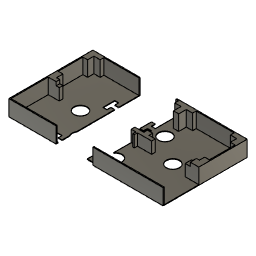
loose_split (Autodesk Fusion 360 design; units mm, degrees)
Autodesk Fusion 360 part; units mm, degrees
note: some values were not read from the file. Chosen so that the rebuilt part matches the saved one: which face or edge a step refers to. Set by a fixed rule: which sketch regions a step uses.
(part 1 of 2)
sketch "スケッチ1" plane through (0, 0, 0) normal (0, 0, 1) x (1, 0, 0)
  line L0 (0, 0) -> (224, 0)
  line L1 (224, 0) -> (224, 158)
  line L2 (224, 158) -> (0, 158)
  line L3 (0, 158) -> (0, 0)
  dimension "d1" = 224
  dimension "d2" = 158
  constraint horizontal L0
  constraint vertical L1
  constraint horizontal L2
  constraint vertical L3
  constraint coincident L0.start L3.end
  measures "d1" distance of L0.start L0.end
  measures "d2" distance of L0.start L2.end
extrude "押し出し1" add sketch "スケッチ1" along normal blind 30 makes body 1
sketch "スケッチ2" plane through (0, 0, 30) normal (0, 0, 1) x (-1, 0, 0)
  line L0 (0, -158) -> (0, 0)
  line L1 (0, 0) -> (-224, 0)
  line L2 (-224, 0) -> (-224, -158)
  line L3 (-224, -158) -> (0, -158)
  line L4 (0, 0) -> (-2, 0)
  line L5 (-2, 0) -> (-2, -2)
  line L6 (-2, -2) -> (0, -2)
  line L7 (0, -2) -> (0, 0)
  line L8 (-224, -158) -> (-222, -158)
  line L9 (-222, -158) -> (-222, -156)
  line L10 (-222, -156) -> (-224, -156)
  line L11 (-224, -156) -> (-224, -158)
  dimension "d5" = 2
  dimension "d6" = 2
  dimension "d7" = 2
  dimension "d8" = 2
  constraint horizontal L4
  constraint vertical L5
  constraint horizontal L6
  constraint vertical L7
  constraint coincident L0.end L1.start
  constraint horizontal L8
  constraint vertical L9
  constraint horizontal L10
  constraint vertical L11
  constraint coincident L2.end L3.start
  measures "d5" distance of L0.end L4.end
  measures "d6" distance of L0.end L6.end
  measures "d7" distance of L2.end L8.end
  measures "d8" distance of L2.end L10.end
sketch "スケッチ3" plane through (0, 0, 30) normal (0, 0, 1) x (-1, 0, 0)
  line L0 (-2, -2) -> (-222, -2)
  line L1 (-222, -2) -> (-222, -156)
  line L2 (-222, -156) -> (-2, -156)
  line L3 (-2, -156) -> (-2, -2)
  point P0 (-2, -2)
  point P1 (-222, -156)
  constraint horizontal L0
  constraint vertical L1
  constraint horizontal L2
  constraint vertical L3
  constraint coincident P1 L1.end
  constraint coincident P0 L0.start
extrude "押し出し2" cut sketch "スケッチ3" against normal blind 28 bodies 1
sketch "スケッチ4" plane through (0, 0, 2) normal (0, 0, 1) x (-1, 0, 0)
  line L0 (-2, -156) -> (-2, -2)
  line L1 (-2, -2) -> (-222, -2)
  line L2 (-222, -2) -> (-222, -156)
  line L3 (-222, -156) -> (-2, -156)
sketch "スケッチ14" plane through (0, 0, 30) normal (0, 0, 1) x (-1, 0, 0)
  line L0 (-222, -2) -> (-2, -2)
  line L1 (-2, -2) -> (-2, -156)
  line L2 (-2, -156) -> (-222, -156)
  line L3 (-222, -156) -> (-222, -2)
  line L4 (0, -158) -> (0, 0)
  line L5 (0, 0) -> (-224, 0)
  line L6 (-224, 0) -> (-224, -158)
  line L7 (-224, -158) -> (0, -158)
sketch "スケッチ15" plane through (0, 0, 30) normal (0, 0, 1) x (-1, 0, 0)
  line L0 (-224, -2) -> (-99, -2)
  line L1 (-99, -2) -> (-99, -66)
  line L2 (-99, -66) -> (-224, -66)
  line L3 (-224, -66) -> (-224, -2)
  line L4 (-224, 0) -> (-224, -158)
  dimension "d41" = 125
  dimension "d42" = 64
  constraint horizontal L0
  constraint vertical L1
  constraint horizontal L2
  constraint vertical L3
  constraint coincident L0.start L4
  measures "d41" distance of L0.start L0.end
  measures "d42" distance of L0.start L2.end
extrude "押し出し10" cut sketch "スケッチ15" against normal blind 29 bodies 1
sketch "スケッチ16" plane through (0, 0, 30) normal (0, 0, 1) x (-1, 0, 0)
  line L0 (-2, -2) -> (-99, -2)
  line L1 (-99, -2) -> (-99, -73)
  line L2 (-99, -73) -> (-2, -73)
  line L3 (-2, -73) -> (-2, -2)
  point P0 (-2, -2)
  dimension "d45" = 71
  constraint horizontal L0
  constraint vertical L1
  constraint horizontal L2
  constraint vertical L3
  constraint coincident P0 L0.start
  measures "d45" distance of P0 L2.end
extrude "押し出し11" add 1 faces at (182.3333, 23.3333, 1) along direction (0, 0, 1) blind 1 on bodies 1 bodies 1
sketch "スケッチ17" plane through (0, 0, 30) normal (0, 0, 1) x (1, 0, 0)
  line L0 (2, 156) -> (11, 156)
  line L1 (11, 156) -> (11, 147)
  line L2 (11, 147) -> (2, 147)
  line L3 (2, 147) -> (2, 156)
  line L4 (11, 147) -> (107, 147)
  line L5 (107, 147) -> (107, 76)
  line L6 (107, 76) -> (11, 76)
  line L7 (11, 76) -> (11, 147)
  line L8 (222, 156) -> (213, 156)
  line L9 (213, 156) -> (213, 147)
  line L10 (213, 147) -> (222, 147)
  line L11 (222, 147) -> (222, 156)
  line L12 (213, 147) -> (117, 147)
  line L13 (117, 147) -> (117, 76)
  line L14 (117, 76) -> (213, 76)
  line L15 (213, 76) -> (213, 147)
  point P0 (2, 156)
  point P1 (222, 156)
  dimension "d48" = 9
  dimension "d49" = 9
  dimension "d50" = 96
  dimension "d51" = 71
  dimension "d52" = 9
  dimension "d53" = 9
  dimension "d54" = 96
  dimension "d55" = 71
  constraint horizontal L0
  constraint vertical L1
  constraint horizontal L2
  constraint vertical L3
  constraint coincident P0 L0.start
  constraint horizontal L4
  constraint vertical L5
  constraint horizontal L6
  constraint vertical L7
  constraint horizontal L8
  constraint vertical L9
  constraint horizontal L10
  constraint vertical L11
  constraint coincident P1 L8.start
  constraint horizontal L12
  constraint vertical L13
  constraint horizontal L14
  constraint vertical L15
  measures "d48" distance of P0 L0.end
  measures "d49" distance of P0 L2.end
  measures "d50" distance of L1.end L4.end
  measures "d51" distance of L1.end L6.end
  measures "d52" distance of P1 L8.end
  measures "d53" distance of P1 L10.end
  measures "d54" distance of L9.end L12.end
  measures "d55" distance of L9.end L14.end
sketch "スケッチ18" plane through (0, 0, 30) normal (0, 0, 1) x (-1, 0, 0)
  line L0 (-11, -147) -> (-2, -147)
  line L1 (-2, -147) -> (-2, -138)
  line L2 (-2, -138) -> (-11, -138)
  line L3 (-11, -138) -> (-11, -147)
  line L4 (-11, -147) -> (-20, -147)
  line L5 (-20, -147) -> (-20, -156)
  line L6 (-20, -156) -> (-11, -156)
  line L7 (-11, -156) -> (-11, -147)
  point P0 (-11, -147)
  dimension "d56" = 9
  dimension "d57" = 9
  dimension "d58" = 9
  constraint horizontal L0
  constraint vertical L1
  constraint horizontal L2
  constraint vertical L3
  constraint coincident P0 L0.start
  constraint horizontal L4
  constraint vertical L5
  constraint horizontal L6
  constraint vertical L7
  measures "d56" distance of P0 L0.end
  measures "d57" distance of P0 L2.end
  measures "d58" distance of P0 L6.end
extrude "押し出し12" add sketch "スケッチ17" sketch "スケッチ18" against normal blind 28 contours L0 L1 L2 L3 of sketch 2 bodies 1
sketch "スケッチ19" plane through (0, 0, 2) normal (0, 0, 1) x (-1, 0, 0)
  line L0 (-213, -147) -> (-222, -147)
  line L1 (-222, -147) -> (-222, -138)
  line L2 (-222, -138) -> (-213, -138)
  line L3 (-213, -138) -> (-213, -147)
  line L4 (-213, -147) -> (-204, -147)
  line L5 (-204, -147) -> (-204, -156)
  line L6 (-204, -156) -> (-213, -156)
  line L7 (-213, -156) -> (-213, -147)
  point P0 (-213, -147)
  dimension "d61" = 9
  dimension "d62" = 9
  dimension "d63" = 9
  dimension "d64" = 9
  constraint horizontal L0
  constraint vertical L1
  constraint horizontal L2
  constraint vertical L3
  constraint coincident P0 L0.start
  constraint horizontal L4
  constraint vertical L5
  constraint horizontal L6
  constraint vertical L7
  measures "d61" distance of P0 L0.end
  measures "d62" distance of P0 L2.end
  measures "d63" distance of P0 L4.end
  measures "d64" distance of P0 L6.end
extrude "押し出し13" add sketch "スケッチ19" along normal blind 28 separate body makes body 2 at (210, 147, 11.3333)
extrude "押し出し14" add sketch "スケッチ17" against normal blind 28 contours L8 L9 L10 L11 bodies 1 2
sketch "スケッチ20" plane through (0, 0, 2) normal (0, 0, 1) x (-1, 0, 0)
  line L0 (-107, -147) -> (-117, -147)
  line L1 (-117, -147) -> (-117, -138)
  line L2 (-117, -138) -> (-107, -138)
  line L3 (-107, -138) -> (-107, -147)
  line L4 (-107, -147) -> (-98, -147)
  line L5 (-98, -147) -> (-98, -156)
  line L6 (-98, -156) -> (-107, -156)
  line L7 (-107, -156) -> (-107, -147)
  line L8 (-117, -147) -> (-126, -147)
  line L9 (-126, -147) -> (-126, -156)
  line L10 (-126, -156) -> (-117, -156)
  line L11 (-117, -156) -> (-117, -147)
  line L12 (-99, -66) -> (-126, -66)
  line L13 (-126, -66) -> (-126, -76)
  line L14 (-126, -76) -> (-99, -76)
  line L15 (-99, -76) -> (-99, -66)
  line L16 (-107, -76) -> (-117, -76)
  line L17 (-117, -76) -> (-117, -85)
  line L18 (-117, -85) -> (-107, -85)
  line L19 (-107, -85) -> (-107, -76)
  point P0 (-107, -147)
  point P1 (-99, -66)
  point P2 (-107, -76)
  dimension "d69" = 10
  dimension "d70" = 9
  dimension "d71" = 9
  dimension "d72" = 9
  dimension "d73" = 9
  dimension "d74" = 9
  dimension "d75" = 27
  dimension "d76" = 9
  constraint horizontal L0
  constraint vertical L1
  constraint horizontal L2
  constraint vertical L3
  constraint coincident P0 L0.start
  constraint horizontal L4
  constraint vertical L5
  constraint horizontal L6
  constraint vertical L7
  constraint horizontal L8
  constraint vertical L9
  constraint horizontal L10
  constraint vertical L11
  constraint horizontal L12
  constraint vertical L13
  constraint horizontal L14
  constraint vertical L15
  constraint coincident P1 L12.start
  constraint horizontal L16
  constraint vertical L17
  constraint horizontal L18
  constraint vertical L19
  constraint coincident P2 L16.start
  measures "d69" distance of P0 L0.end
  measures "d70" distance of P0 L2.end
  measures "d71" distance of P0 L4.end
  measures "d72" distance of P0 L6.end
  measures "d73" distance of L0.end L8.end
  measures "d74" distance of L0.end L10.end
  measures "d75" distance of P1 L12.end
  measures "d76" distance of P2 L18.end
extrude "押し出し15" add sketch "スケッチ20" along normal blind 28 separate body contours L8 L9 L10 L11 | L0 L1 L2 L3 | L4 L5 L6 L7 makes body 3 at (104, 147, 11.3333)
extrude "押し出し16" add 1 faces at (110.3333, 147, 11.3333) along direction (0, 1, 0) blind 9 on bodies 3 bodies 1 3
extrude "押し出し17" add sketch "スケッチ20" along normal blind 28 contours L12 L13 L14 L15 L16 | L14 L16 L17 L18 L19 bodies 1
sketch "スケッチ21" plane through (0, 0, 2) normal (0, 0, 1) x (-1, 0, 0)
  line L0 (-99, -76) -> (-90, -76)
  line L1 (-90, -76) -> (-90, -73)
  line L2 (-90, -73) -> (-99, -73)
  line L3 (-99, -73) -> (-99, -76)
  point P0 (-99, -76)
  dimension "d83" = 9
  constraint horizontal L0
  constraint vertical L1
  constraint horizontal L2
  constraint vertical L3
  constraint coincident P0 L0.start
  measures "d83" distance of P0 L0.end
extrude "押し出し18" add sketch "スケッチ21" along normal blind 28 bodies 1
sketch "スケッチ22" plane through (0, 0, 2) normal (0, 0, 1) x (-1, 0, 0)
  line L0 (-11, -76) -> (-20, -76)
  line L1 (-20, -76) -> (-20, -73)
  line L2 (-20, -73) -> (-11, -73)
  line L3 (-11, -73) -> (-11, -76)
  line L4 (-11, -73) -> (-2, -73)
  line L5 (-2, -73) -> (-2, -85)
  line L6 (-2, -85) -> (-11, -85)
  line L7 (-11, -85) -> (-11, -73)
  point P0 (-11, -76)
  dimension "d86" = 9
  dimension "d87" = 3
  dimension "d88" = 12
  constraint horizontal L0
  constraint vertical L1
  constraint horizontal L2
  constraint vertical L3
  constraint coincident P0 L0.start
  constraint horizontal L4
  constraint vertical L5
  constraint horizontal L6
  constraint vertical L7
  measures "d86" distance of P0 L0.end
  measures "d87" distance of P0 L2.end
  measures "d88" distance of L2.end L6.end
extrude "押し出し19" add sketch "スケッチ22" along normal blind 28 bodies 1
sketch "スケッチ23" plane through (0, 0, 2) normal (0, 0, 1) x (-1, 0, 0)
  line L0 (-213, -76) -> (-204, -76)
  line L1 (-204, -76) -> (-204, -66)
  line L2 (-204, -66) -> (-213, -66)
  line L3 (-213, -66) -> (-213, -76)
  line L4 (-213, -76) -> (-222, -76)
  line L5 (-222, -76) -> (-222, -85)
  line L6 (-222, -85) -> (-213, -85)
  line L7 (-213, -85) -> (-213, -76)
  line L8 (-213, -76) -> (-222, -76)
  line L9 (-222, -76) -> (-222, -66)
  line L10 (-222, -66) -> (-213, -66)
  line L11 (-213, -66) -> (-213, -76)
  point P0 (-213, -76)
  point P1 (-222, -66)
  dimension "d91" = 9
  dimension "d92" = 9
  dimension "d93" = 9
  constraint horizontal L0
  constraint vertical L1
  constraint horizontal L2
  constraint vertical L3
  constraint coincident P0 L0.start
  constraint horizontal L4
  constraint vertical L5
  constraint horizontal L6
  constraint vertical L7
  constraint horizontal L8
  constraint vertical L9
  constraint horizontal L10
  constraint vertical L11
  constraint coincident P1 L9.end
  measures "d91" distance of P0 L0.end
  measures "d92" distance of P0 L4.end
  measures "d93" distance of P0 L6.end
extrude "押し出し20" add sketch "スケッチ23" along normal blind 28 bodies 1
sketch "スケッチ24" plane through (0, 0, 30) normal (0, 0, 1) x (-1, 0, 0)
  line L0 (-107, -138) -> (-117, -138)
  line L1 (-117, -138) -> (-117, -147)
  line L2 (-117, -147) -> (-126, -147)
  line L3 (-126, -147) -> (-126, -156)
  line L4 (-126, -156) -> (-204, -156)
  line L5 (-204, -156) -> (-204, -147)
  line L6 (-204, -147) -> (-213, -147)
  line L7 (-213, -147) -> (-213, -138)
  line L8 (-213, -138) -> (-222, -138)
  line L9 (-222, -138) -> (-222, -85)
  line L10 (-222, -85) -> (-213, -85)
  line L11 (-213, -85) -> (-213, -76)
  line L12 (-213, -76) -> (-204, -76)
  line L13 (-204, -76) -> (-204, -66)
  line L14 (-204, -66) -> (-224, -66)
  line L15 (-224, -66) -> (-224, -158)
  line L16 (-224, -158) -> (0, -158)
  line L17 (0, -158) -> (0, 0)
  line L18 (0, 0) -> (-224, 0)
  line L19 (-224, 0) -> (-224, -2)
  line L20 (-224, -2) -> (-2, -2)
  line L21 (-2, -2) -> (-2, -73)
  line L22 (-2, -73) -> (-20, -73)
  line L23 (-20, -73) -> (-20, -76)
  line L24 (-20, -76) -> (-11, -76)
  line L25 (-11, -76) -> (-11, -85)
  line L26 (-11, -85) -> (-2, -85)
  line L27 (-2, -85) -> (-2, -138)
  line L28 (-2, -138) -> (-11, -138)
  line L29 (-11, -138) -> (-11, -147)
  line L30 (-11, -147) -> (-20, -147)
  line L31 (-20, -147) -> (-20, -156)
  line L32 (-20, -156) -> (-98, -156)
  line L33 (-98, -156) -> (-98, -147)
  line L34 (-98, -147) -> (-107, -147)
  line L35 (-107, -147) -> (-107, -138)
  line L36 (-2, -156) -> (-222, -156)
  line L37 (-222, -156) -> (-222, -2)
  line L38 (-222, -2) -> (-2, -2)
  line L39 (-2, -2) -> (-2, -156)
  point P0 (-2, -156)
  point P1 (-222, -2)
  constraint horizontal L36
  constraint vertical L37
  constraint horizontal L38
  constraint vertical L39
  constraint coincident P1 L37.end
  constraint coincident P0 L36.start
extrude "押し出し21" cut sketch "スケッチ24" against normal blind 7 contours L0 L1 L2 L3 L33 L34 L35 L36 | L0 L1 L2 L3 L4 L5 L6 L7 L8 L9 L10 L11 L12 L13 L14 L20 L21 L22 L23 L24 L25 L26 L27 L28 L29 L30 L31 L32 L33 L34 L35 L36 L37 L38 L39 | L28 L29 L30 L31 L36 L39 | L5 L6 L7 L8 L36 L37 | L22 L23 L24 L25 L26 L39 | L10 L11 L12 L13 L14 L37 bodies 1
sketch "スケッチ25" plane through (0, 0, 30) normal (0, 0, 1) x (1, 0, 0)
  line L0 (90, 73) -> (85, 73)
  line L1 (85, 73) -> (85, -7.0693)
  line L2 (85, -7.0693) -> (90, -7.0693)
  line L3 (90, -7.0693) -> (90, 73)
  line L4 (90, 73) -> (85, 73)
  line L5 (85, 73) -> (85, 169.9061)
  line L6 (85, 169.9061) -> (90, 169.9061)
  line L7 (90, 169.9061) -> (90, 73)
  point P0 (90, 73)
  dimension "d98" = 5
  dimension "d99" = 5
  constraint horizontal L0
  constraint vertical L1
  constraint horizontal L2
  constraint vertical L3
  constraint coincident P0 L0.start
  constraint horizontal L4
  constraint vertical L5
  constraint horizontal L6
  constraint vertical L7
  measures "d98" distance of P0 L0.end
  measures "d99" distance of P0 L0.end
extrude "押し出し22" cut sketch "スケッチ25" against normal blind 70 bodies 1 makes body 4 at (28.3333, 105.3333, 0)
move_body "移動1" bodies 1 to x (1, 0, 0) y (0, 1, 0) z (0, 0, 1) at (70, 0, 0)
extrude "押し出し23" add 1 faces at (85, 53.3333, 0.6667) along direction (1, 0, 0) blind 5 on bodies 4 bodies 4
sketch "スケッチ26" plane through (0, 0, 2) normal (0, 0, 1) x (-1, 0, 0)
  line L0 (-90, -156) -> (-20, -156)
  line L1 (-20, -156) -> (-20, -147)
  line L2 (-20, -147) -> (-11, -147)
  line L3 (-11, -147) -> (-11, -138)
  line L4 (-11, -138) -> (-2, -138)
  line L5 (-2, -138) -> (-2, -85)
  line L6 (-2, -85) -> (-11, -85)
  line L7 (-11, -85) -> (-11, -76)
  line L8 (-11, -76) -> (-20, -76)
  line L9 (-20, -76) -> (-20, -73)
  line L10 (-20, -73) -> (-2, -73)
  line L11 (-2, -73) -> (-2, -2)
  line L12 (-2, -2) -> (-90, -2)
  line L13 (-90, -2) -> (-90, -156)
  line L14 (-160, -2) -> (-90, -2)
  line L15 (-90, -2) -> (-90, -29)
  line L16 (-90, -29) -> (-160, -29)
  line L17 (-160, -29) -> (-160, -2)
  line L18 (-90, -29) -> (-160, -29)
  line L19 (-160, -29) -> (-160, -39)
  line L20 (-160, -39) -> (-90, -39)
  line L21 (-90, -39) -> (-90, -29)
  line L22 (-90, -39) -> (-80, -39)
  line L23 (-80, -39) -> (-80, -29)
  line L24 (-80, -29) -> (-90, -29)
  line L25 (-90, -29) -> (-90, -39)
  line L26 (-160, -29) -> (-169.6, -29)
  line L27 (-169.6, -29) -> (-169.6, -34)
  line L28 (-169.6, -34) -> (-160, -34)
  line L29 (-160, -34) -> (-160, -29)
  line L30 (-160, -34) -> (-169.6, -34)
  line L31 (-169.6, -34) -> (-169.6, -38.8)
  line L32 (-169.6, -38.8) -> (-160, -38.8)
  line L33 (-160, -38.8) -> (-160, -34)
  line L34 (-160, -34) -> (-169.6, -34)
  line L35 (-169.6, -34) -> (-169.6, -29.5)
  line L36 (-169.6, -29.5) -> (-160, -29.5)
  line L37 (-160, -29.5) -> (-160, -34)
  point P0 (-160, -2)
  dimension "d104" = 27
  dimension "d105" = 10
  dimension "d106" = 10
  dimension "d107" = 10
  dimension "d108" = 9.6
  dimension "d109" = 5
  dimension "d110" = 9.6
  dimension "d111" = 4.8
  dimension "d112" = 9.6
  dimension "d113" = 4.5
  constraint horizontal L14
  constraint vertical L15
  constraint horizontal L16
  constraint vertical L17
  constraint coincident L13 L15.end
  constraint coincident P0 L14.start
  constraint horizontal L18
  constraint vertical L19
  constraint horizontal L20
  constraint vertical L21
  constraint horizontal L22
  constraint vertical L23
  constraint horizontal L24
  constraint vertical L25
  constraint horizontal L26
  constraint vertical L27
  constraint horizontal L28
  constraint vertical L29
  constraint horizontal L30
  constraint vertical L31
  constraint horizontal L32
  constraint vertical L33
  constraint horizontal L34
  constraint vertical L35
  constraint horizontal L36
  constraint vertical L37
  measures "d104" distance of P0 L16.end
  measures "d105" distance of L15.end L20.end
  measures "d106" distance of L20.end L22.end
  measures "d107" distance of L20.end L15.end
  measures "d108" distance of L16.end L26.end
  measures "d109" distance of L16.end L28.end
  measures "d110" distance of L28.end L27.end
  measures "d111" distance of L28.end L32.end
  measures "d112" distance of L28.end L27.end
  measures "d113" distance of L28.end L36.end
extrude "押し出し24" cut sketch "スケッチ26" against normal blind 3 contours L19 L28 L30 L31 L32 L33 L34 | L19 L27 L28 L29 L30 L34 L35 L36 L37 bodies 1
extrude "押し出し25" cut sketch "スケッチ26" against normal blind 17 contours L13 L21 L22 L23 L24 L25 bodies 4
extrude "押し出し26" add 1 faces at (80, 35.6667, 0.6667) along direction (1, 0, 0) blind 20 on bodies 4 bodies 4
sketch "スケッチ27" plane through (0, 0, 2) normal (0, 0, 1) x (-1, 0, 0)
  line L0 (-169.6, -29.5) -> (-160, -29.5)
  line L1 (-160, -29.5) -> (-160, -2)
  line L2 (-160, -2) -> (-294, -2)
  line L3 (-294, -2) -> (-294, -66)
  line L4 (-294, -66) -> (-274, -66)
  line L5 (-274, -66) -> (-274, -76)
  line L6 (-274, -76) -> (-283, -76)
  line L7 (-283, -76) -> (-283, -85)
  line L8 (-283, -85) -> (-292, -85)
  line L9 (-292, -85) -> (-292, -138)
  line L10 (-292, -138) -> (-283, -138)
  line L11 (-283, -138) -> (-283, -147)
  line L12 (-283, -147) -> (-274, -147)
  line L13 (-274, -147) -> (-274, -156)
  line L14 (-274, -156) -> (-196, -156)
  line L15 (-196, -156) -> (-196, -147)
  line L16 (-196, -147) -> (-187, -147)
  line L17 (-187, -147) -> (-187, -138)
  line L18 (-187, -138) -> (-177, -138)
  line L19 (-177, -138) -> (-177, -147)
  line L20 (-177, -147) -> (-168, -147)
  line L21 (-168, -147) -> (-168, -156)
  line L22 (-168, -156) -> (-160, -156)
  line L23 (-160, -156) -> (-160, -76)
  line L24 (-160, -76) -> (-177, -76)
  line L25 (-177, -76) -> (-177, -85)
  line L26 (-177, -85) -> (-187, -85)
  line L27 (-187, -85) -> (-187, -76)
  line L28 (-187, -76) -> (-196, -76)
  line L29 (-196, -76) -> (-196, -66)
  line L30 (-196, -66) -> (-169, -66)
  line L31 (-169, -66) -> (-169, -73)
  line L32 (-169, -73) -> (-160, -73)
  line L33 (-160, -73) -> (-160, -38.8)
  line L34 (-160, -38.8) -> (-169.6, -38.8)
  line L35 (-169.6, -38.8) -> (-169.6, -29.5)
  line L36 (-177, -138) -> (-160, -138)
  line L37 (-160, -138) -> (-160, -116.5)
  line L38 (-160, -116.5) -> (-177, -116.5)
  line L39 (-177, -116.5) -> (-177, -138)
  line L40 (-160, -116.5) -> (-170, -116.5)
  line L41 (-170, -116.5) -> (-170, -106.5)
  line L42 (-170, -106.5) -> (-160, -106.5)
  line L43 (-160, -106.5) -> (-160, -116.5)
  dimension "d120" = 21.5
  dimension "d121" = 10
  dimension "d122" = 10
  constraint horizontal L36
  constraint vertical L37
  constraint horizontal L38
  constraint vertical L39
  constraint coincident L18.end L19.start
  constraint horizontal L40
  constraint vertical L41
  constraint horizontal L42
  constraint vertical L43
  measures "d120" distance of L18.end L38.end
  measures "d121" distance of L37.end L40.end
  measures "d122" distance of L37.end L42.end
extrude "押し出し27" cut sketch "スケッチ27" against normal blind 31 contours L23 L38 L40 L41 L42 L43 bodies 1
extrude "押し出し28" add 1 faces at (170, 113.1667, 0.6667) along direction (-1, 0, 0) blind 20 on bodies 1 bodies 1
sketch "スケッチ28" plane through (0, 0, 2) normal (0, 0, 1) x (-1, 0, 0)
  line L0 (-160, -106.5) -> (-160, -76)
  line L1 (-160, -76) -> (-177, -76)
  line L2 (-177, -76) -> (-177, -85)
  line L3 (-177, -85) -> (-187, -85)
  line L4 (-187, -85) -> (-187, -76)
  line L5 (-187, -76) -> (-196, -76)
  line L6 (-196, -76) -> (-196, -66)
  line L7 (-196, -66) -> (-169, -66)
  line L8 (-169, -66) -> (-169, -73)
  line L9 (-169, -73) -> (-160, -73)
  line L10 (-160, -73) -> (-160, -38.8)
  line L11 (-160, -38.8) -> (-169.6, -38.8)
  line L12 (-169.6, -38.8) -> (-169.6, -29.5)
  line L13 (-169.6, -29.5) -> (-160, -29.5)
  line L14 (-160, -29.5) -> (-160, -2)
  line L15 (-160, -2) -> (-294, -2)
  line L16 (-294, -2) -> (-294, -66)
  line L17 (-294, -66) -> (-274, -66)
  line L18 (-274, -66) -> (-274, -76)
  line L19 (-274, -76) -> (-283, -76)
  line L20 (-283, -76) -> (-283, -85)
  line L21 (-283, -85) -> (-292, -85)
  line L22 (-292, -85) -> (-292, -138)
  line L23 (-292, -138) -> (-283, -138)
  line L24 (-283, -138) -> (-283, -147)
  line L25 (-283, -147) -> (-274, -147)
  line L26 (-274, -147) -> (-274, -156)
  line L27 (-274, -156) -> (-196, -156)
  line L28 (-196, -156) -> (-196, -147)
  line L29 (-196, -147) -> (-187, -147)
  line L30 (-187, -147) -> (-187, -138)
  line L31 (-187, -138) -> (-177, -138)
  line L32 (-177, -138) -> (-177, -147)
  line L33 (-177, -147) -> (-168, -147)
  line L34 (-168, -147) -> (-168, -156)
  line L35 (-168, -156) -> (-160, -156)
  line L36 (-160, -156) -> (-160, -116.5)
  line L37 (-160, -116.5) -> (-150, -116.5)
  line L38 (-150, -116.5) -> (-150, -106.5)
  line L39 (-150, -106.5) -> (-160, -106.5)
  line L40 (-150, -116.5) -> (-90, -116.5)
  line L41 (-90, -116.5) -> (-90, -111.5)
  line L42 (-90, -111.5) -> (-150, -111.5)
  line L43 (-150, -111.5) -> (-150, -116.5)
  dimension "d127" = 5
  constraint horizontal L40
  constraint vertical L41
  constraint horizontal L42
  constraint vertical L43
  constraint coincident L37.end L38.start
  measures "d127" distance of L37.end L42.end
sketch "スケッチ29" plane through (0, 0, 2) normal (0, 0, 1) x (-1, 0, 0)
  line L0 (-90, -111.5) -> (-80.4, -111.5)
  line L1 (-80.4, -111.5) -> (-80.4, -106.7)
  line L2 (-80.4, -106.7) -> (-90, -106.7)
  line L3 (-90, -106.7) -> (-90, -111.5)
  line L4 (-90, -111.5) -> (-80.4, -111.5)
  line L5 (-80.4, -111.5) -> (-80.4, -116.3)
  line L6 (-80.4, -116.3) -> (-90, -116.3)
  line L7 (-90, -116.3) -> (-90, -111.5)
  point P0 (-90, -111.5)
  dimension "d128" = 9.6
  dimension "d129" = 4.8
  dimension "d130" = 4.8
  constraint horizontal L0
  constraint vertical L1
  constraint horizontal L2
  constraint vertical L3
  constraint coincident P0 L0.start
  constraint horizontal L4
  constraint vertical L5
  constraint horizontal L6
  constraint vertical L7
  measures "d128" distance of P0 L0.end
  measures "d129" distance of P0 L2.end
  measures "d130" distance of P0 L6.end
extrude "押し出し29" cut sketch "スケッチ29" against normal blind 10 bodies 4
sketch "スケッチ30" plane through (0, 38.8, 0) normal (0, -1, 0) x (1, 0, 0)
  line L0 (160, 0) -> (169.6, 0)
  line L1 (169.6, 0) -> (169.6, 2)
  line L2 (169.6, 2) -> (160, 2)
  line L3 (160, 2) -> (160, 0)
extrude "押し出し30" cut 1 faces at (86.8, 116.3, 0.6667) along direction (0, 1, 0) blind 0.75 on bodies 4 bodies 4
extrude "押し出し31" cut 1 faces at (86.8, 106.7, 0.6667) along direction (0, -1, 0) blind 0.75 on bodies 4 bodies 4
extrude "押し出し32" add 1 faces at (86.8, 105.95, 0.6667) along direction (0, 1, 0) blind 0.2 on bodies 4 bodies 4
extrude "押し出し33" add 1 faces at (86.8, 117.05, 0.6667) along direction (0, -1, 0) blind 0.2 on bodies 4 bodies 4
extrude "押し出し34" cut 1 faces at (86.8, 116.85, 0.6667) along direction (0, 1, 0) blind 0.25 on bodies 4 bodies 4
extrude "押し出し35" cut 1 faces at (86.8, 106.15, 0.6667) along direction (0, -1, 0) blind 0.25 on bodies 4 bodies 4
extrude "押し出し36" cut 1 faces at (96.6667, 29, 1.3333) along direction (0, 1, 0) blind 0.95 on bodies 4 bodies 4
extrude "押し出し37" cut 1 faces at (93.3333, 39, 1.3333) along direction (0, -1, 0) blind 0.95 on bodies 4 bodies 4
sketch "スケッチ31" plane through (0, 0, 2) normal (0, 0, 1) x (-1, 0, 0)
  line L0 (-160, -106.5) -> (-160, -76)
  line L1 (-160, -76) -> (-177, -76)
  line L2 (-177, -76) -> (-177, -85)
  line L3 (-177, -85) -> (-187, -85)
  line L4 (-187, -85) -> (-187, -76)
  line L5 (-187, -76) -> (-196, -76)
  line L6 (-196, -76) -> (-196, -66)
  line L7 (-196, -66) -> (-169, -66)
  line L8 (-169, -66) -> (-169, -73)
  line L9 (-169, -73) -> (-160, -73)
  line L10 (-160, -73) -> (-160, -38.8)
  line L11 (-160, -38.8) -> (-169.6, -38.8)
  line L12 (-169.6, -38.8) -> (-169.6, -29.5)
  line L13 (-169.6, -29.5) -> (-160, -29.5)
  line L14 (-160, -29.5) -> (-160, -2)
  line L15 (-160, -2) -> (-294, -2)
  line L16 (-294, -2) -> (-294, -66)
  line L17 (-294, -66) -> (-274, -66)
  line L18 (-274, -66) -> (-274, -76)
  line L19 (-274, -76) -> (-283, -76)
  line L20 (-283, -76) -> (-283, -85)
  line L21 (-283, -85) -> (-292, -85)
  line L22 (-292, -85) -> (-292, -138)
  line L23 (-292, -138) -> (-283, -138)
  line L24 (-283, -138) -> (-283, -147)
  line L25 (-283, -147) -> (-274, -147)
  line L26 (-274, -147) -> (-274, -156)
  line L27 (-274, -156) -> (-196, -156)
  line L28 (-196, -156) -> (-196, -147)
  line L29 (-196, -147) -> (-187, -147)
  line L30 (-187, -147) -> (-187, -138)
  line L31 (-187, -138) -> (-177, -138)
  line L32 (-177, -138) -> (-177, -147)
  line L33 (-177, -147) -> (-168, -147)
  line L34 (-168, -147) -> (-168, -156)
  line L35 (-168, -156) -> (-160, -156)
  line L36 (-160, -156) -> (-160, -116.5)
  line L37 (-160, -116.5) -> (-150, -116.5)
  line L38 (-150, -116.5) -> (-150, -106.5)
  line L39 (-150, -106.5) -> (-160, -106.5)
  line L40 (-187, -76) -> (-177.2801, -76)
  line L41 (-177.2801, -76) -> (-177.2801, -2)
  line L42 (-177.2801, -2) -> (-187, -2)
  line L43 (-187, -2) -> (-187, -76)
  line L44 (-187, -2) -> (-283, -2)
  line L45 (-283, -2) -> (-283, -73)
  line L46 (-283, -73) -> (-187, -73)
  line L47 (-187, -73) -> (-187, -2)
  dimension "d149" = 96
  dimension "d150" = 71
  constraint horizontal L40
  constraint vertical L41
  constraint horizontal L42
  constraint vertical L43
  constraint coincident L15 L41.end
  constraint coincident L4.end L5.start
  constraint horizontal L44
  constraint vertical L45
  constraint horizontal L46
  constraint vertical L47
  measures "d149" distance of L42.end L44.end
  measures "d150" distance of L42.end L46.end
extrude "押し出し38" cut sketch "スケッチ31" along normal blind 25 contours L6 L7 L43 L46 L47 | L17 L18 L45 L46 bodies 1
extrude "押し出し39" cut 4 faces at (14, 147, 16) (174, 147, 16) (190, 147, 9) (280, 147, 9) along direction (0, 1, 0) blind 2 on bodies 1 4 bodies 1 4
extrude "押し出し40" add 4 faces at (14, 76, 9) (171.3333, 76, 16) (280, 76, 16) (193, 76, 16) along direction (0, 1, 0) blind 2 on bodies 1 4 bodies 4 1
extrude "押し出し41" add 6 faces at (5, 147.6667, 23) (5, 78.6667, 23) (177.6667, 70, 23) (183.6667, 153.6667, 23) (289, 147.6667, 23) (289, 74.6667, 23) along direction (0, 0, 1) blind 7 on bodies 1 4 bodies 4 1
sketch "スケッチ32" plane through (0, 0, 30) normal (0, 0, 1) x (-1, 0, 0)
  line L0 (-90, -158) -> (0, -158)
  line L1 (0, -158) -> (0, 0)
  line L2 (0, 0) -> (-90, 0)
  line L3 (-90, 0) -> (-90, -2)
  line L4 (-90, -2) -> (-2, -2)
  line L5 (-2, -2) -> (-2, -73)
  line L6 (-2, -73) -> (-20, -73)
  line L7 (-20, -73) -> (-20, -78)
  line L8 (-20, -78) -> (-11, -78)
  line L9 (-11, -78) -> (-11, -85)
  line L10 (-11, -85) -> (-2, -85)
  line L11 (-2, -85) -> (-2, -138)
  line L12 (-2, -138) -> (-11, -138)
  line L13 (-11, -138) -> (-11, -149)
  line L14 (-11, -149) -> (-20, -149)
  line L15 (-20, -149) -> (-20, -156)
  line L16 (-20, -156) -> (-90, -156)
  line L17 (-90, -156) -> (-90, -158)
sketch "スケッチ33" plane through (0, 0, 30) normal (0, 0, 1) x (-1, 0, 0)
  line L0 (-17, -156) -> (-278.5, -156)
  line L1 (-278.5, -156) -> (-278.5, -41.8867)
  line L2 (-278.5, -41.8867) -> (-17, -41.8867)
  line L3 (-17, -41.8867) -> (-17, -156)
  dimension "d159" = 261.5
  constraint horizontal L0
  constraint vertical L1
  constraint horizontal L2
  constraint vertical L3
  measures "d159" distance of L0.start L0.end
extrude "押し出し42" cut sketch "スケッチ33" against normal blind 7 bodies 1 4
extrude "押し出し43" cut sketch "スケッチ30" against normal blind 0.95 bodies 1
extrude "押し出し44" cut 1 faces at (166.4, 29.5, 1.3333) along direction (0, -1, 0) blind 0.95 on bodies 1 bodies 1
extrude "押し出し45" add 1 faces at (93.3333, 38.05, 1.3333) along direction (0, 1, 0) blind 0.95 on bodies 4 bodies 4
extrude "押し出し46" add 1 faces at (96.6667, 29.95, 1.3333) along direction (0, -1, 0) blind 0.95 on bodies 4 bodies 4
extrude "押し出し47" cut 1 faces at (150, 113.1667, 0.6667) along direction (1, 0, 0) blind 0.3 on bodies 1 bodies 1
extrude "押し出し48" cut 1 faces at (100, 32.3333, 1.3333) along direction (-1, 0, 0) blind 0.3 on bodies 4 bodies 4
extrude "押し出し49" add 1 faces at (18, 153.6667, 23) along direction (0, 0, 1) blind 7 on bodies 4 bodies 4
extrude "押し出し50" add 1 faces at (183.6667, 153.6667, 23) along direction (0, 0, 1) blind 7 on bodies 1 bodies 1
extrude "押し出し51" add 1 faces at (277, 151.3333, 23) along direction (0, 0, 1) blind 7 on bodies 1 bodies 1
extrude "押し出し52" cut 2 faces at (26.8, 87.9667, 0) (252.5333, 65.9167, 0) along direction (0, 0, 1) blind 1 on bodies 1 4 bodies 1 4
extrude "押し出し53" add 3 faces at (177.6667, 70, 23) (18, 76.3333, 23) (277, 74.6667, 23) along direction (0, 0, 1) blind 1 on bodies 1 4 bodies 1 4
extrude "押し出し54" add 1 faces at (278.5, 76.3333, 28) along direction (-1, 0, 0) blind 1 on bodies 1 bodies 1
extrude "押し出し55" add 1 faces at (183.6667, 138, 11.3333) along direction (0, -1, 0) blind 1.5 on bodies 1 bodies 1
extrude "押し出し56" cut 1 faces at (187, 68.3333, 9.3333) along direction (-1, 0, 0) blind 15 on bodies 1 bodies 1
extrude "押し出し57" add 1 faces at (283, 68.3333, 11.3333) along direction (-1, 0, 0) blind 15 on bodies 1 bodies 1
sketch "スケッチ34" plane through (0, 73, 0) normal (0, 1, 0) x (-1, 0, 0)
  line L0 (-277.5, 30) -> (-277.5, 24)
  line L1 (-277.5, 24) -> (-274, 24)
  line L2 (-274, 24) -> (-274, 2)
  line L3 (-274, 2) -> (-268, 2)
  line L4 (-268, 2) -> (-268, 30)
  line L5 (-268, 30) -> (-277.5, 30)
sketch "スケッチ35" plane through (272.75, 73, 16) normal (0, 1, 0) x (-1, 0, 0)
  line L0 (-4.75, 8) -> (4.75, 8)
  line L1 (4.75, 8) -> (4.75, 14)
  line L2 (4.75, 14) -> (-4.75, 14)
  line L3 (-4.75, 14) -> (-4.75, 8)
  point P0 (-4.75, 8)
  point P1 (4.75, 14)
  constraint horizontal L0
  constraint vertical L1
  constraint horizontal L2
  constraint vertical L3
  constraint coincident P1 L1.end
  constraint coincident P0 L0.start
extrude "押し出し58" cut sketch "スケッチ35" against normal blind 13 bodies 1
sketch "スケッチ5" plane through (0, 0, 2) normal (0, 0, 1) x (-1, 0, 0)
  line L0 (-2, -156) -> (-73, -156)
  line L1 (-73, -156) -> (-73, -60)
  line L2 (-73, -60) -> (-2, -60)
  line L3 (-2, -60) -> (-2, -156)
  line L4 (-222, -156) -> (-151, -156)
  line L5 (-151, -156) -> (-151, -60)
  line L6 (-151, -60) -> (-222, -60)
  line L7 (-222, -60) -> (-222, -156)
  point P0 (-2, -156)
  point P1 (-222, -156)
  dimension "d11" = 71
  dimension "d12" = 96
  dimension "d13" = 71
  dimension "d14" = 96
  constraint horizontal L0
  constraint vertical L1
  constraint horizontal L2
  constraint vertical L3
  constraint coincident P0 L0.start
  constraint horizontal L4
  constraint vertical L5
  constraint horizontal L6
  constraint vertical L7
  constraint coincident P1 L4.start
  measures "d11" distance of P0 L0.end
  measures "d12" distance of P0 L2.end
  measures "d13" distance of P1 L4.end
  measures "d14" distance of P1 L6.end
extrude "押し出し59" add sketch "スケッチ32" 2 faces at (289.6667, 148.3333, 30) (248.6667, 0.6667, 30) along normal blind 1 on bodies 1 bodies 1 4
extrude "押し出し60" cut 1 faces at (19, 74.6667, 30) along direction (0, 0, 1) blind 2 on bodies 4 bodies 4
sketch "スケッチ6" plane through (0, 0, 2) normal (0, 0, 1) x (-1, 0, 0)
  line L0 (-73, -156) -> (-76.5, -156)
  line L1 (-76.5, -156) -> (-76.5, -60)
  line L2 (-76.5, -60) -> (-73, -60)
  line L3 (-73, -60) -> (-73, -156)
  line L4 (-151, -156) -> (-147.5, -156)
  line L5 (-147.5, -156) -> (-147.5, -60)
  line L6 (-147.5, -60) -> (-151, -60)
  line L7 (-151, -60) -> (-151, -156)
  point P0 (-73, -156)
  point P1 (-151, -156)
  dimension "d15" = 3.5
  dimension "d16" = 96
  dimension "d17" = 3.5
  dimension "d18" = 96
  constraint horizontal L0
  constraint vertical L1
  constraint horizontal L2
  constraint vertical L3
  constraint coincident P0 L0.start
  constraint horizontal L4
  constraint vertical L5
  constraint horizontal L6
  constraint vertical L7
  constraint coincident P1 L4.start
  measures "d15" distance of P0 L0.end
  measures "d16" distance of P0 L2.end
  measures "d17" distance of P1 L4.end
  measures "d18" distance of P1 L6.end
extrude "押し出し61" add 1 faces at (96.4667, 29, 1.6667) along direction (0, -1, 0) blind 0.2 on bodies 4 bodies 4
extrude "押し出し62" add 1 faces at (93.2333, 39, 1.6667) along direction (0, 1, 0) blind 0.2 on bodies 4 bodies 4
extrude "押し出し63" add 1 faces at (153.5333, 116.5, 1.6667) along direction (0, 1, 0) blind 0.2 on bodies 1 bodies 1
extrude "押し出し64" add 1 faces at (153.5333, 106.5, 1.6667) along direction (0, -1, 0) blind 0.2 on bodies 1 bodies 1
sketch "スケッチ36" plane through (0, 0, 2) normal (0, 0, 1) x (-1, 0, 0)
  line L0 (-294, -66) -> (-268, -66)
  line L1 (-268, -66) -> (-268, -73)
  line L2 (-268, -73) -> (-274, -73)
  line L3 (-274, -73) -> (-274, -78)
  line L4 (-274, -78) -> (-283, -78)
  line L5 (-283, -78) -> (-283, -85)
  line L6 (-283, -85) -> (-292, -85)
  line L7 (-292, -85) -> (-292, -138)
  line L8 (-292, -138) -> (-283, -138)
  line L9 (-283, -138) -> (-283, -149)
  line L10 (-283, -149) -> (-274, -149)
  line L11 (-274, -149) -> (-274, -156)
  line L12 (-274, -156) -> (-196, -156)
  line L13 (-196, -156) -> (-196, -149)
  line L14 (-196, -149) -> (-187, -149)
  line L15 (-187, -149) -> (-187, -136.5)
  line L16 (-187, -136.5) -> (-177, -136.5)
  line L17 (-177, -136.5) -> (-177, -149)
  line L18 (-177, -149) -> (-168, -149)
  line L19 (-168, -149) -> (-168, -156)
  line L20 (-168, -156) -> (-160, -156)
  line L21 (-160, -156) -> (-160, -116.7)
  line L22 (-160, -116.7) -> (-150.3, -116.7)
  line L23 (-150.3, -116.7) -> (-150.3, -106.3)
  line L24 (-150.3, -106.3) -> (-160, -106.3)
  line L25 (-160, -106.3) -> (-160, -78)
  line L26 (-160, -78) -> (-177, -78)
  line L27 (-177, -78) -> (-177, -85)
  line L28 (-177, -85) -> (-187, -85)
  line L29 (-187, -85) -> (-187, -78)
  line L30 (-187, -78) -> (-196, -78)
  line L31 (-196, -78) -> (-196, -73)
  line L32 (-196, -73) -> (-172, -73)
  line L33 (-172, -73) -> (-172, -66)
  line L34 (-172, -66) -> (-169, -66)
  line L35 (-169, -66) -> (-169, -73)
  line L36 (-169, -73) -> (-160, -73)
  line L37 (-160, -73) -> (-160, -39.75)
  line L38 (-160, -39.75) -> (-169.6, -39.75)
  line L39 (-169.6, -39.75) -> (-169.6, -28.55)
  line L40 (-169.6, -28.55) -> (-160, -28.55)
  line L41 (-160, -28.55) -> (-160, -2)
  line L42 (-160, -2) -> (-294, -2)
  line L43 (-294, -2) -> (-294, -66)
  line L44 (-196, -78) -> (-207.6595, -78)
  line L45 (-207.6595, -78) -> (-207.6595, -75.5)
  line L46 (-207.6595, -75.5) -> (-196, -75.5)
  line L47 (-196, -75.5) -> (-196, -78)
  line L48 (-187, -78) -> (-235, -78)
  line L49 (-235, -78) -> (-235, -75.5)
  line L50 (-235, -75.5) -> (-187, -75.5)
  line L51 (-187, -75.5) -> (-187, -78)
  circle A0 centre (-235, -75.5) radius 12.5
  dimension "d206" = 48
  dimension "d207" = 2.5
  dimension "d208" = 25
  constraint horizontal L44
  constraint vertical L45
  constraint horizontal L46
  constraint vertical L47
  constraint coincident L30.end L31.start
  constraint horizontal L48
  constraint vertical L49
  constraint horizontal L50
  constraint vertical L51
  constraint coincident L29.end L30.start
  constraint coincident L49.end L50.start
  measures "d206" distance of L29.end L48.end
  measures "d207" distance of L29.end L50.end
  measures "d208" diameter of A0
extrude "押し出し65" cut sketch "スケッチ36" against normal blind 10 contours L48 L49 L50 A0 | L48 L49 L50 A0 bodies 1
sketch "スケッチ37" plane through (0, 0, 2) normal (0, 0, 1) x (-1, 0, 0)
  line L0 (-99.7, -28.8) -> (-99.7, -39.2)
  line L1 (-99.7, -39.2) -> (-90, -39.2)
  line L2 (-90, -39.2) -> (-90, -105.9)
  line L3 (-90, -105.9) -> (-80.4, -105.9)
  line L4 (-80.4, -105.9) -> (-80.4, -117.1)
  line L5 (-80.4, -117.1) -> (-90, -117.1)
  line L6 (-90, -117.1) -> (-90, -156)
  line L7 (-90, -156) -> (-20, -156)
  line L8 (-20, -156) -> (-20, -149)
  line L9 (-20, -149) -> (-11, -149)
  line L10 (-11, -149) -> (-11, -138)
  line L11 (-11, -138) -> (-2, -138)
  line L12 (-2, -138) -> (-2, -85)
  line L13 (-2, -85) -> (-11, -85)
  line L14 (-11, -85) -> (-11, -78)
  line L15 (-11, -78) -> (-20, -78)
  line L16 (-20, -78) -> (-20, -73)
  line L17 (-20, -73) -> (-2, -73)
  line L18 (-2, -73) -> (-2, -2)
  line L19 (-2, -2) -> (-90, -2)
  line L20 (-90, -2) -> (-90, -28.8)
  line L21 (-90, -28.8) -> (-99.7, -28.8)
  line L22 (-11, -78) -> (-59, -78)
  line L23 (-59, -78) -> (-59, -75.5)
  line L24 (-59, -75.5) -> (-11, -75.5)
  line L25 (-11, -75.5) -> (-11, -78)
  circle A0 centre (-59, -75.5) radius 12.5
  dimension "d211" = 48
  dimension "d212" = 2.5
  dimension "d213" = 25
  constraint horizontal L22
  constraint vertical L23
  constraint horizontal L24
  constraint vertical L25
  constraint coincident L14.end L15.start
  constraint coincident L23.end L24.start
  measures "d211" distance of L14.end L22.end
  measures "d212" distance of L14.end L24.end
  measures "d213" diameter of A0
extrude "押し出し66" cut sketch "スケッチ37" against normal blind 7 contours L22 L23 L24 A0 | L22 L23 L24 A0 bodies 4
sketch "スケッチ38" plane through (0, 0, 2) normal (0, 0, 1) x (-1, 0, 0)
  circle A0 centre (-235, -75.5) radius 12.5
  line L0 (-294, -66) -> (-268, -66)
  line L1 (-268, -66) -> (-268, -73)
  line L2 (-268, -73) -> (-274, -73)
  line L3 (-274, -73) -> (-274, -78)
  line L4 (-274, -78) -> (-283, -78)
  line L5 (-283, -78) -> (-283, -85)
  line L6 (-283, -85) -> (-292, -85)
  line L7 (-292, -85) -> (-292, -138)
  line L8 (-292, -138) -> (-283, -138)
  line L9 (-283, -138) -> (-283, -149)
  line L10 (-283, -149) -> (-274, -149)
  line L11 (-274, -149) -> (-274, -156)
  line L12 (-274, -156) -> (-196, -156)
  line L13 (-196, -156) -> (-196, -149)
  line L14 (-196, -149) -> (-187, -149)
  line L15 (-187, -149) -> (-187, -136.5)
  line L16 (-187, -136.5) -> (-177, -136.5)
  line L17 (-177, -136.5) -> (-177, -149)
  line L18 (-177, -149) -> (-168, -149)
  line L19 (-168, -149) -> (-168, -156)
  line L20 (-168, -156) -> (-160, -156)
  line L21 (-160, -156) -> (-160, -116.7)
  line L22 (-160, -116.7) -> (-150.3, -116.7)
  line L23 (-150.3, -116.7) -> (-150.3, -106.3)
  line L24 (-150.3, -106.3) -> (-160, -106.3)
  line L25 (-160, -106.3) -> (-160, -78)
  line L26 (-160, -78) -> (-177, -78)
  line L27 (-177, -78) -> (-177, -85)
  line L28 (-177, -85) -> (-187, -85)
  line L29 (-187, -85) -> (-187, -78)
  line L30 (-187, -78) -> (-196, -78)
  line L31 (-196, -78) -> (-196, -73)
  line L32 (-196, -73) -> (-172, -73)
  line L33 (-172, -73) -> (-172, -66)
  line L34 (-172, -66) -> (-169, -66)
  line L35 (-169, -66) -> (-169, -73)
  line L36 (-169, -73) -> (-160, -73)
  line L37 (-160, -73) -> (-160, -39.75)
  line L38 (-160, -39.75) -> (-169.6, -39.75)
  line L39 (-169.6, -39.75) -> (-169.6, -28.55)
  line L40 (-169.6, -28.55) -> (-160, -28.55)
  line L41 (-160, -28.55) -> (-160, -2)
  line L42 (-160, -2) -> (-294, -2)
  line L43 (-294, -2) -> (-294, -66)
  line L44 (-187, -149) -> (-182, -149)
  line L45 (-182, -149) -> (-182, -113.5)
  line L46 (-182, -113.5) -> (-187, -113.5)
  line L47 (-187, -113.5) -> (-187, -149)
  circle A1 centre (-182, -113.5) radius 12.5
  dimension "d216" = 5
  dimension "d217" = 35.5
  dimension "d218" = 25
  constraint horizontal L44
  constraint vertical L45
  constraint horizontal L46
  constraint vertical L47
  constraint coincident L14.end L15.start
  constraint coincident L45.end L46.start
  measures "d216" distance of L14.end L44.end
  measures "d217" distance of L14.end L46.end
  measures "d218" diameter of A1
extrude "押し出し67" cut sketch "スケッチ38" against normal blind 12 contours L45 L46 L47 A1 | L45 L46 L47 A1 bodies 1
sketch "スケッチ39" plane through (0, 0, 0) normal (0, 0, 1) x (1, 0, 0)
  line L0 (90, 39.2) -> (160, 39.2)
  line L1 (160, 39.2) -> (160, 28.8)
  line L2 (160, 28.8) -> (90, 28.8)
  line L3 (90, 28.8) -> (90, 39.2)
  point P0 (90, 39.2)
  dimension "d221" = 70
  constraint horizontal L0
  constraint vertical L1
  constraint horizontal L2
  constraint vertical L3
  constraint coincident P0 L0.start
  measures "d221" distance of P0 L0.end
extrude "押し出し68" cut 1 faces at (150.3, 113.2333, 1.6667) along direction (1, 0, 0) blind 0.2 on bodies 1 bodies 1
extrude "押し出し69" cut 1 faces at (96.4667, 28.8, 1.6667) along direction (0, 1, 0) blind 11 on bodies 4 bodies 4
sketch "スケッチ40" plane through (0, 0, 0) normal (0, 0, 1) x (1, 0, 0)
  line L0 (160, 39.75) -> (150.5, 39.75)
  line L1 (150.5, 39.75) -> (150.5, 34.15)
  line L2 (150.5, 34.15) -> (160, 34.15)
  line L3 (160, 34.15) -> (160, 39.75)
  line L4 (160, 34.15) -> (150.5, 34.15)
  line L5 (150.5, 34.15) -> (150.5, 28.95)
  line L6 (150.5, 28.95) -> (160, 28.95)
  line L7 (160, 28.95) -> (160, 34.15)
  line L8 (160, 34.15) -> (150.5, 34.15)
  line L9 (150.5, 34.15) -> (150.5, 39.35)
  line L10 (150.5, 39.35) -> (160, 39.35)
  line L11 (160, 39.35) -> (160, 34.15)
  point P0 (160, 39.75)
  dimension "d226" = 9.5
  dimension "d227" = 5.6
  dimension "d228" = 9.5
  dimension "d229" = 5.2
  dimension "d230" = 5.2
  constraint horizontal L0
  constraint vertical L1
  constraint horizontal L2
  constraint vertical L3
  constraint coincident P0 L0.start
  constraint horizontal L4
  constraint vertical L5
  constraint horizontal L6
  constraint vertical L7
  constraint horizontal L8
  constraint vertical L9
  constraint horizontal L10
  constraint vertical L11
  measures "d226" distance of P0 L0.end
  measures "d227" distance of P0 L2.end
  measures "d228" distance of L2.end L1.end
  measures "d229" distance of L2.end L6.end
  measures "d230" distance of L2.end L10.end
extrude "押し出し70" add sketch "スケッチ40" along normal blind 1 separate body contours L1 L2 L3 L4 L8 L9 L10 L11 | L2 L4 L5 L6 L7 L8 makes body 5
extrude "押し出し71" add 1 faces at (153.6667, 37.6167, 1) along direction (0, 0, 1) blind 1 on bodies 5 bodies 5
extrude "押し出し72" cut 1 faces at (156.8333, 32.4167, 0) along direction (0, 0, 1) blind 1 on bodies 5 bodies 5
extrude "押し出し73" add 1 faces at (166.4, 39.75, 1.3333) along direction (0, -1, 0) blind 13 on bodies 1 bodies 1 5
sketch "スケッチ41" plane through (0, 0, 2) normal (0, 0, 1) x (-1, 0, 0)
  circle A0 centre (-235, -75.5) radius 12.5
  circle A1 centre (-182, -113.5) radius 12.5
  line L0 (-160, -28.95) -> (-160, -2)
  line L1 (-160, -2) -> (-294, -2)
  line L2 (-294, -2) -> (-294, -66)
  line L3 (-294, -66) -> (-268, -66)
  line L4 (-268, -66) -> (-268, -73)
  line L5 (-268, -73) -> (-274, -73)
  line L6 (-274, -73) -> (-274, -78)
  line L7 (-274, -78) -> (-283, -78)
  line L8 (-283, -78) -> (-283, -85)
  line L9 (-283, -85) -> (-292, -85)
  line L10 (-292, -85) -> (-292, -138)
  line L11 (-292, -138) -> (-283, -138)
  line L12 (-283, -138) -> (-283, -149)
  line L13 (-283, -149) -> (-274, -149)
  line L14 (-274, -149) -> (-274, -156)
  line L15 (-274, -156) -> (-196, -156)
  line L16 (-196, -156) -> (-196, -149)
  line L17 (-196, -149) -> (-187, -149)
  line L18 (-187, -149) -> (-187, -136.5)
  line L19 (-187, -136.5) -> (-177, -136.5)
  line L20 (-177, -136.5) -> (-177, -149)
  line L21 (-177, -149) -> (-168, -149)
  line L22 (-168, -149) -> (-168, -156)
  line L23 (-168, -156) -> (-160, -156)
  line L24 (-160, -156) -> (-160, -116.7)
  line L25 (-160, -116.7) -> (-150.5, -116.7)
  line L26 (-150.5, -116.7) -> (-150.5, -106.3)
  line L27 (-150.5, -106.3) -> (-160, -106.3)
  line L28 (-160, -106.3) -> (-160, -78)
  line L29 (-160, -78) -> (-177, -78)
  line L30 (-177, -78) -> (-177, -85)
  line L31 (-177, -85) -> (-187, -85)
  line L32 (-187, -85) -> (-187, -78)
  line L33 (-187, -78) -> (-196, -78)
  line L34 (-196, -78) -> (-196, -73)
  line L35 (-196, -73) -> (-172, -73)
  line L36 (-172, -73) -> (-172, -66)
  line L37 (-172, -66) -> (-169, -66)
  line L38 (-169, -66) -> (-169, -73)
  line L39 (-169, -73) -> (-160, -73)
  line L40 (-160, -73) -> (-160, -39.35)
  line L41 (-160, -39.35) -> (-150.5, -39.35)
  line L42 (-150.5, -39.35) -> (-150.5, -28.95)
  line L43 (-150.5, -28.95) -> (-160, -28.95)
  line L44 (-160, -39.35) -> (-90, -39.35)
  line L45 (-90, -39.35) -> (-90, -34.15)
  line L46 (-90, -34.15) -> (-160, -34.15)
  line L47 (-160, -34.15) -> (-160, -39.35)
  dimension "d239" = 70
  dimension "d240" = 5.2
  constraint horizontal L44
  constraint vertical L45
  constraint horizontal L46
  constraint vertical L47
  constraint coincident L40.end L41.start
  measures "d239" distance of L40.end L44.end
  measures "d240" distance of L40.end L46.end
sketch "スケッチ42" plane through (0, 0, 2) normal (0, 0, 1) x (-1, 0, 0)
  line L0 (-90, -2) -> (-90, -105.9)
  line L1 (-90, -105.9) -> (-80.4, -105.9)
  line L2 (-80.4, -105.9) -> (-80.4, -117.1)
  line L3 (-80.4, -117.1) -> (-90, -117.1)
  line L4 (-90, -117.1) -> (-90, -156)
  line L5 (-90, -156) -> (-20, -156)
  line L6 (-20, -156) -> (-20, -149)
  line L7 (-20, -149) -> (-11, -149)
  line L8 (-11, -149) -> (-11, -138)
  line L9 (-11, -138) -> (-2, -138)
  line L10 (-2, -138) -> (-2, -85)
  line L11 (-2, -85) -> (-11, -85)
  line L12 (-11, -85) -> (-11, -78)
  line L13 (-11, -78) -> (-20, -78)
  line L14 (-20, -78) -> (-20, -73)
  line L15 (-20, -73) -> (-2, -73)
  line L16 (-2, -73) -> (-2, -2)
  line L17 (-2, -2) -> (-90, -2)
  circle A0 centre (-59, -75.5) radius 12.5
  line L18 (-90, -34.15) -> (-80.4, -34.15)
  line L19 (-80.4, -34.15) -> (-80.4, -39.75)
  line L20 (-80.4, -39.75) -> (-90, -39.75)
  line L21 (-90, -39.75) -> (-90, -34.15)
  line L22 (-90, -34.15) -> (-80.4, -34.15)
  line L23 (-80.4, -34.15) -> (-80.4, -28.55)
  line L24 (-80.4, -28.55) -> (-90, -28.55)
  line L25 (-90, -28.55) -> (-90, -34.15)
  point P0 (-90, -34.15)
  dimension "d241" = 9.6
  dimension "d242" = 5.6
  dimension "d243" = 5.6
  constraint horizontal L18
  constraint vertical L19
  constraint horizontal L20
  constraint vertical L21
  constraint coincident P0 L18.start
  constraint horizontal L22
  constraint vertical L23
  constraint horizontal L24
  constraint vertical L25
  measures "d241" distance of P0 L18.end
  measures "d242" distance of P0 L20.end
  measures "d243" distance of P0 L24.end
extrude "押し出し74" cut sketch "スケッチ42" against normal blind 60 contours L0 L18 L22 L23 L24 L25 | L0 L18 L19 L20 L21 L22 bodies 4